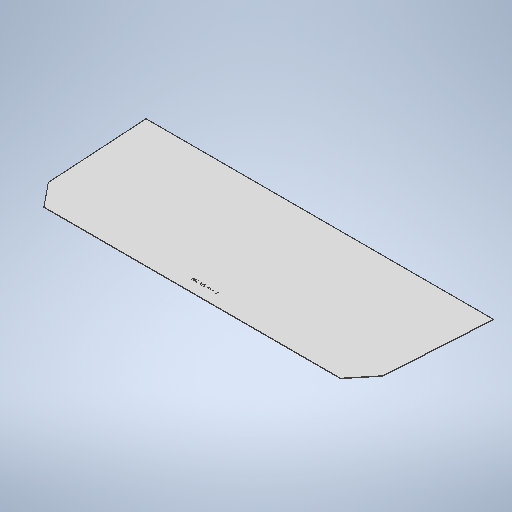
# Autodesk Inventor part: MSC 075 face 2
Saved by Autodesk Inventor 2025 (Build 290162010, 162A)
## iProperties
Created: 2024-06-16
Part Number: MSC 075 face 2
Material: AISI304
Document SubType Name: Sheet Metal
Designer: admin
Density: 8 g/cm^3
Sheet Metal Rule: AISI304 2mm Die16
Appearance: Default
Stock Number: МОО 075 морда 2
Flat Pattern Width: 58.1083 cm
Flat Pattern Length: 158.284 cm
Flat Pattern Area: 9197.64 cm^2
Sheet Metal Width: 581,083 mm
Sheet Metal Length: 1582,844 mm
Sheet Metal Area: 919763,945 mm^2
Author: admin
Autodesk Inventor part; units mm, degrees
ref_plane "YZ Plane" through (0, 0, 0) normal (1, 0, 0) x (0, 1, 0)
ref_plane "XZ Plane" through (0, 0, 0) normal (0, 1, 0) x (-1, 0, 0)
ref_plane "XY Plane" through (0, 0, 0) normal (0, 0, 1) x (1, 0, 0)
sketch "Sketch1" plane through (0, 0, 0) normal (0, 0, 1) x (1, 0, 0)
  line L0 (791.422, 0) -> (791.422, -581.0831) construction
  line L1 (791.422, -581.0831) -> (0, -581.0831)
  line L2 (751.2327, -472.4176) -> (662.7706, -581.0831) construction
  ellipse E0 centre (-10250, 902.1234) end of major axis (-10250, -13526.5434) minor radius 11053 (753.0938, -467.4569) -> (781.265, -2.2899) ccw construction
  line L3 (791.422, 0) -> (762.706, -474.1635)
  line L4 (675.6653, -581.0831) -> (791.422, -438.8891)
  line L5 (753.0938, -467.4569) -> (763.0755, -468.0614) construction
  line L6 (781.265, -2.2899) -> (791.2468, -2.8944) construction
  line L7 (0, -581.0831) -> (0, 0)
  line L8 (0, 0) -> (791.422, 0)
  dimension "d3" = 10
  dimension "d4" = 10
  dimension "d5" = 10
  measures "d3" distance between parallel lines of L4 L2
  measures "d4" distance of L5.start L5.end
  measures "d5" distance of L6.start L6.end
extrude "Plate1" add sketch "Sketch1" along normal blind 2
mirror "Mirror1" about plane through (0, 0, 0) normal (1, 0, 0) of "Plate1"
sketch "Sketch2" plane through (0, 0, 2) normal (0, 0, 1) x (1, 0, 0)
  line L0 (-55, -531.0831) -> (-55, -519.0831) construction
  line L1 (-55, -519.0831) -> (55, -519.0831) construction
  line L2 (55, -519.0831) -> (55, -531.0831) construction
  line L3 (55, -531.0831) -> (-55, -531.0831) construction
  line L4 (-675.6653, -581.0831) -> (675.6653, -581.0831) projected
  point P0 (0, 0)
  point P1 (0, -531.0831)
  point P2 (0, -581.0831)
  dimension "d6" = 12
  dimension "d7" = 110
  dimension "d8" = 50
  constraints: 2 midpoint, 1 parallel, 1 vertical alignment, 2 other
  measures "d6" distance of L1.end L2.end
  measures "d7" distance between parallel lines of L0 L2
  measures "d8" distance between parallel lines of L4 L3
mark "Mark1"
equation "\"d2\" = Thickness"
equation "\"BendReliefWidth\" = Thickness"
equation "\"BendReliefDepth\" = 0.5 * Thickness"
equation "\"CornerReliefSize\" = 4 * Thickness"
equation "\"MinimumRemnant\" = 2 * Thickness"
equation "\"TransitionRadius\" = BendRadius"
equation "\"JacobiRadiusSize\" = BendRadius"
equation "\"GapSize\" = Thickness"
equation "\"Thickness\" = 2"
equation "\"BendRadius\" = 2.75"
body "Solid1"
